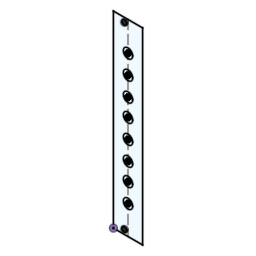
FU-CADETV-SCALER v5 (Autodesk Fusion 360 design; units mm, degrees)
Autodesk Fusion 360 part; units mm, degrees
sketch "Sketch1" plane through (0, 0, 0) normal (0, 1, 0) x (1, 0, 0)
  line L0 (0, 0) -> (20, 0)
  line L1 (20, 0) -> (20, -128.5)
  line L2 (20, -128.5) -> (0, -128.5)
  line L3 (0, -128.5) -> (0, 0)
  line L4 (10, -128.5) -> (10, 0) construction
  circle A0 centre (10, -108.5) radius 3.16
  circle A1 centre (10, -95.5) radius 3.16
  circle A2 centre (7.5, -125.5) radius 1.6
  circle A3 centre (10, -70.5) radius 3.16
  circle A4 centre (10, -57.5) radius 3.16
  circle A5 centre (10, -82.5) radius 3.16
  circle A6 centre (10, -44.5) radius 3.16
  circle A7 centre (7.5, -3) radius 1.6
  circle A8 centre (10, -32.5) radius 3.16
  circle A9 centre (10, -19.5) radius 3.16
  dimension "d1" = 20
  dimension "d2" = 128.5
  dimension "d3" = 6.32
  dimension "d4" = 20
  dimension "d5" = 6.32
  dimension "d6" = 33
  dimension "d7" = 3.2
  dimension "d8" = 7.5
  dimension "d9" = 6.32
  dimension "d10" = 58
  dimension "d11" = 6.32
  dimension "d12" = 6.32
  dimension "d13" = 6.32
  dimension "d14" = 71
  dimension "d15" = 46
  dimension "d16" = 84
  dimension "d17" = 3
  dimension "d18" = 3.2
  dimension "d19" = 3
  dimension "d20" = 7.5
  dimension "d21" = 6.32
  dimension "d22" = 96
  dimension "d23" = 6.32
  dimension "d24" = 109
  dimension "d27" = 13
  dimension "d28" = 13
  dimension "d29" = 13
  dimension "d30" = 12
  dimension "d31" = 13
  dimension "d32" = 13
  dimension "d33" = 12
  constraint horizontal L0
  constraint vertical L1
  constraint horizontal L2
  constraint vertical L3
  constraint coincident L0.start L3.end
  constraint midpoint L2 L4.start
  constraint midpoint L0 L4.end
  constraint coincident L4 A0.centre
  constraint coincident L4 A1.centre
  constraint coincident L4 A5.centre
  constraint coincident L4 A3.centre
  constraint coincident L4 A4.centre
  constraint coincident L4 A6.centre
  constraint coincident L4 A8.centre
  constraint coincident L4 A9.centre
  measures "d1" distance of L1.end L2.end
  measures "d2" distance of L0.end L1.end
  measures "d3" diameter of A0
  measures "d4" distance of L4.start A0.centre
  measures "d5" diameter of A1
  measures "d6" distance of L2 A1.centre
  measures "d7" diameter of A2
  measures "d8" distance of L3 A2.centre
  measures "d9" diameter of A3
  measures "d10" distance of L2 A3.centre
  measures "d11" diameter of A4
  measures "d12" diameter of A5
  measures "d13" diameter of A6
  measures "d14" distance of L2 A4.centre
  measures "d15" distance of L2 A5.centre
  measures "d16" distance of L2 A6.centre
  measures "d17" distance of L2 A2.centre
  measures "d18" diameter of A7
  measures "d19" distance of L0 A7.centre
  measures "d20" distance of L3 A7.centre
  measures "d21" diameter of A8
  measures "d22" distance of L2 A8.centre
  measures "d23" diameter of A9
  measures "d24" distance of L2 A9.centre
  measures "d27" distance of A6.centre A4.centre
  measures "d28" distance of A8.centre A9.centre
  measures "d29" distance of A0.centre A1.centre
  measures "d30" distance of A3.centre A5.centre
  measures "d31" distance of A1.centre A5.centre
  measures "d32" distance of A3.centre A4.centre
  measures "d33" distance of A6.centre A8.centre
extrude "Extrude1" add sketch "Sketch1" along normal blind 2
hidden bodies 1
equation "d5 = d3"
equation "d9 = d3"
equation "d11 = d3"
equation "d12 = d3"
equation "d13 = d3"
equation "d21 = d3"
equation "d23 = d3"
